Autodesk Inventor part; units mm, degrees
(part 2 of 2)
  arc A608 (10.5835, 25.1123) -> (10.4066, 24.8539) centre (14.8434, 22.0065) ccw
  arc A609 (10.8252, 25.4234) -> (10.5835, 25.1123) centre (15.7615, 21.3378) ccw
  arc A610 (11.147, 25.7878) -> (10.8252, 25.4234) centre (16.6706, 20.5861) ccw
  arc A611 (9.9958, 26.1618) -> (9.6113, 26.2702) centre (4.2393, 6.4866) ccw
  arc A612 (10.0419, 25.6779) -> (9.9958, 26.1618) centre (2.4697, 25.2002) ccw
  arc A613 (10.0547, 25.2841) -> (10.0419, 25.6779) centre (3.647, 25.2741) ccw
  arc A614 (10.4066, 24.8539) -> (10.0459, 24.9711) centre (4.2393, 6.4866) ccw
  arc A615 (10.0459, 24.9711) -> (10.0547, 25.2841) centre (4.7827, 25.2754) ccw
  arc A616 (9.1026, 25.5526) -> (8.9465, 25.2811) centre (13.5931, 22.7906) ccw
  arc A617 (9.3192, 25.8817) -> (9.1026, 25.5526) centre (14.5608, 22.1961) ccw
  arc A618 (9.6113, 26.2702) -> (9.3192, 25.8817) centre (15.526, 21.5179) ccw
  arc A619 (8.4344, 26.5528) -> (8.0426, 26.6307) centre (4.2393, 6.4866) ccw
  arc A620 (8.5183, 26.074) -> (8.4344, 26.5528) centre (1.0069, 25.0037) ccw
  arc A621 (8.5619, 25.6824) -> (8.5183, 26.074) centre (2.1747, 25.1697) ccw
  arc A622 (8.9465, 25.2811) -> (8.5777, 25.3697) centre (4.2393, 6.4866) ccw
  arc A623 (8.5777, 25.3697) -> (8.5619, 25.6824) centre (3.3069, 25.2601) ccw
  arc A624 (7.5917, 25.8754) -> (7.4574, 25.5925) centre (12.285, 23.4742) ccw
  arc A625 (7.7818, 26.2205) -> (7.5917, 25.8754) centre (13.2964, 22.9575) ccw
  arc A626 (8.0426, 26.6307) -> (7.7818, 26.2205) centre (14.3119, 22.3571) ccw
  arc A627 (6.8471, 26.8201) -> (6.4504, 26.867) centre (4.2393, 6.4866) ccw
  arc A628 (6.9683, 26.3493) -> (6.8471, 26.8201) centre (-0.436, 24.693) ccw
  arc A629 (7.0425, 25.9624) -> (6.9683, 26.3493) centre (0.7152, 24.9501) ccw
  arc A630 (7.4574, 25.5925) -> (7.0828, 25.6518) centre (4.2393, 6.4866) ccw
  arc A631 (7.0828, 25.6518) -> (7.0425, 25.9624) centre (1.8368, 25.1291) ccw
  arc A632 (6.0601, 26.0787) -> (5.9484, 25.7861) centre (10.9274, 24.0531) ccw
  arc A633 (6.2226, 26.4376) -> (6.0601, 26.0787) centre (11.9762, 23.6173) ccw
  arc A634 (6.4504, 26.867) -> (6.2226, 26.4376) centre (13.0356, 23.0985) ccw
  arc A635 (5.2437, 26.962) -> (4.8445, 26.9777) centre (4.2393, 6.4866) ccw
  arc A636 (5.4015, 26.5022) -> (5.2437, 26.962) centre (-1.85, 24.27) ccw
  arc A637 (5.5058, 26.1223) -> (5.4015, 26.5022) centre (-0.7225, 24.6167) ccw
  arc A638 (5.9484, 25.7861) -> (5.5703, 25.8158) centre (4.2393, 6.4866) ccw
  arc A639 (5.5703, 25.8158) -> (5.5058, 26.1223) centre (0.3816, 24.8831) ccw
  circle A640 centre (-6.2776, 14.9509) radius 1.5
  circle A641 centre (-6.2776, 14.9509) radius 3.5
  circle A642 centre (-4.225, -4.0303) radius 3.5
  circle A643 centre (-4.225, -4.0303) radius 1.5
  circle A644 centre (14.7563, -1.9776) radius 3.5
  circle A645 centre (14.7563, -1.9776) radius 1.5
  circle A646 centre (12.7036, 17.0036) radius 3.5
  circle A647 centre (12.7036, 17.0036) radius 1.5
  line L0 (-2.9801, 19.468) -> (-3.0512, 19.5957)
  circle A648 centre (4.2393, 6.4866) radius 5
  circle A649 centre (4.2393, 6.4866) radius 5.6
  circle A650 centre (4.2393, 6.4866) radius 18.25
  point P0 (0, 0)
  point P1 (4.2393, 28.9866)
  point P2 (2.474, 28.9173)
  point P3 (0.7195, 28.7096)
  point P4 (-1.0132, 28.3649)
  point P5 (-2.7136, 27.8854)
  point P6 (-4.3711, 27.2739)
  point P7 (-5.9755, 26.5343)
  point P8 (-7.5169, 25.671)
  point P9 (-8.9859, 24.6895)
  point P10 (-10.3733, 23.5958)
  point P11 (-11.6706, 22.3965)
  point P12 (-12.8698, 21.0992)
  point P13 (-13.9636, 19.7118)
  point P14 (-14.9451, 18.2428)
  point P15 (-15.8083, 16.7014)
  point P16 (-16.548, 15.097)
  point P17 (-17.1595, 13.4395)
  point P18 (-17.639, 11.7391)
  point P19 (-17.9837, 10.0064)
  point P20 (-18.1913, 8.252)
  point P21 (-18.2607, 6.4866)
  point P22 (-18.1913, 4.7213)
  point P23 (-17.9837, 2.9668)
  point P24 (-17.639, 1.2341)
  point P25 (-17.1595, -0.4663)
  point P26 (-16.548, -2.1238)
  point P27 (-15.8083, -3.7282)
  point P28 (-14.9451, -5.2696)
  point P29 (-13.9636, -6.7385)
  point P30 (-12.8698, -8.126)
  point P31 (-11.6706, -9.4233)
  point P32 (-10.3733, -10.6225)
  point P33 (-8.9859, -11.7163)
  point P34 (-7.5169, -12.6978)
  point P35 (-5.9755, -13.561)
  point P36 (-4.3711, -14.3007)
  point P37 (-2.7136, -14.9121)
  point P38 (-1.0132, -15.3917)
  point P39 (0.7195, -15.7364)
  point P40 (2.474, -15.944)
  point P41 (4.2393, -16.0134)
  point P42 (6.0046, -15.944)
  point P43 (7.7591, -15.7364)
  point P44 (9.4918, -15.3917)
  point P45 (11.1922, -14.9121)
  point P46 (12.8497, -14.3007)
  point P47 (14.4541, -13.561)
  point P48 (15.9955, -12.6978)
  point P49 (17.4645, -11.7163)
  point P50 (18.8519, -10.6225)
  point P51 (20.1492, -9.4233)
  point P52 (21.3484, -8.126)
  point P53 (22.4422, -6.7385)
  point P54 (23.4237, -5.2696)
  point P55 (24.287, -3.7282)
  point P56 (25.0266, -2.1238)
  point P57 (25.6381, -0.4663)
  point P58 (26.1176, 1.2341)
  point P59 (26.4623, 2.9668)
  point P60 (26.6699, 4.7213)
  point P61 (26.7393, 6.4866)
  point P62 (26.6699, 8.252)
  point P63 (26.4623, 10.0064)
  point P64 (26.1176, 11.7391)
  point P65 (25.6381, 13.4395)
  point P66 (25.0266, 15.097)
  point P67 (24.287, 16.7014)
  point P68 (23.4237, 18.2428)
  point P69 (22.4422, 19.7118)
  point P70 (21.3484, 21.0992)
  point P71 (20.1492, 22.3965)
  point P72 (18.8519, 23.5958)
  point P73 (17.4645, 24.6895)
  point P74 (15.9955, 25.671)
  point P75 (14.4541, 26.5343)
  point P76 (12.8497, 27.2739)
  point P77 (11.1922, 27.8854)
  point P78 (9.4918, 28.3649)
  point P79 (7.7591, 28.7096)
  point P80 (6.0046, 28.9173)
  point P81 (23.6134, 6.6762)
  point P82 (23.9112, 6.7638)
  point P83 (24.2822, 6.8975)
  point P84 (24.7304, 7.0918)
  point P85 (24.7147, 7.491)
  point P86 (24.2526, 7.6495)
  point P87 (23.8723, 7.7538)
  point P88 (23.5685, 7.8177)
  point P89 (23.5388, 8.1957)
  point P90 (23.8288, 8.3064)
  point P91 (24.1882, 8.4688)
  point P92 (24.6197, 8.6977)
  point P93 (24.5728, 9.0944)
  point P94 (24.0997, 9.2162)
  point P95 (23.7123, 9.2902)
  point P96 (23.4045, 9.3301)
  point P97 (23.3452, 9.7047)
  point P98 (23.6256, 9.8377)
  point P99 (23.9711, 10.0279)
  point P100 (24.3834, 10.2899)
  point P101 (24.3055, 10.6817)
  point P102 (23.8243, 10.766)
  point P103 (23.4323, 10.8094)
  point P104 (23.1223, 10.825)
  point P105 (23.0338, 11.1938)
  point P106 (23.3029, 11.3484)
  point P107 (23.6325, 11.5651)
  point P108 (24.0229, 11.8587)
  point P109 (23.9145, 12.2431)
  point P110 (23.4282, 12.2894)
  point P111 (23.034, 12.302)
  point P112 (22.7237, 12.2932)
  point P113 (22.6065, 12.6539)
  point P114 (22.8627, 12.8292)
  point P115 (23.1742, 13.071)
  point P116 (23.5404, 13.3943)
  point P117 (23.4022, 13.7691)
  point P118 (22.9138, 13.7771)
  point P119 (22.5198, 13.7587)
  point P120 (22.2112, 13.7256)
  point P121 (22.0661, 14.076)
  point P122 (22.3077, 14.2708)
  point P123 (22.5993, 14.5363)
  point P124 (22.939, 14.8874)
  point P125 (22.7717, 15.2501)
  point P126 (22.2842, 15.2198)
  point P127 (21.8929, 15.1705)
  point P128 (21.5878, 15.1133)
  point P129 (21.4156, 15.4512)
  point P130 (21.6413, 15.6644)
  point P131 (21.9111, 15.952)
  point P132 (22.2222, 16.3286)
  point P133 (22.027, 16.6771)
  point P134 (21.5434, 16.6086)
  point P135 (21.1571, 16.5288)
  point P136 (20.8575, 16.4479)
  point P137 (20.6593, 16.7712)
  point P138 (20.8675, 17.0015)
  point P139 (21.114, 17.3094)
  point P140 (21.3946, 17.7092)
  point P141 (21.1727, 18.0413)
  point P142 (20.6959, 17.9351)
  point P143 (20.3171, 17.8252)
  point P144 (20.0247, 17.721)
  point P145 (19.8018, 18.0278)
  point P146 (19.9913, 18.2737)
  point P147 (20.2128, 18.6)
  point P148 (20.4612, 19.0206)
  point P149 (20.2139, 19.3343)
  point P150 (19.7469, 19.191)
  point P151 (19.3779, 19.0517)
  point P152 (19.0946, 18.9249)
  point P153 (18.8483, 19.2133)
  point P154 (19.0179, 19.4732)
  point P155 (19.2132, 19.8159)
  point P156 (19.4278, 20.2547)
  point P157 (19.1566, 20.548)
  point P158 (18.7023, 20.3685)
  point P159 (18.3454, 20.2008)
  point P160 (18.0729, 20.0521)
  point P161 (17.8048, 20.3202)
  point P162 (17.9535, 20.5927)
  point P163 (18.1212, 20.9496)
  point P164 (18.3007, 21.4039)
  point P165 (18.0074, 21.6751)
  point P166 (17.5686, 21.4605)
  point P167 (17.2259, 21.2652)
  point P168 (16.966, 21.0956)
  point P169 (16.6776, 21.3419)
  point P170 (16.8044, 21.6252)
  point P171 (16.9436, 21.9942)
  point P172 (17.087, 22.4612)
  point P173 (16.7733, 22.7085)
  point P174 (16.3527, 22.4601)
  point P175 (16.0264, 22.2386)
  point P176 (15.7805, 22.0491)
  point P177 (15.4737, 22.272)
  point P178 (15.5779, 22.5644)
  point P179 (15.6878, 22.9432)
  point P180 (15.794, 23.42)
  point P181 (15.4619, 23.6419)
  point P182 (15.0621, 23.3613)
  point P183 (14.7541, 23.1148)
  point P184 (14.5239, 22.9067)
  point P185 (14.2006, 23.1048)
  point P186 (14.2815, 23.4045)
  point P187 (14.3613, 23.7907)
  point P188 (14.4298, 24.2743)
  point P189 (14.0813, 24.4695)
  point P190 (13.7047, 24.1584)
  point P191 (13.4171, 23.8886)
  point P192 (13.2039, 23.663)
  point P193 (12.866, 23.8351)
  point P194 (12.9232, 24.1402)
  point P195 (12.9724, 24.5315)
  point P196 (13.0028, 25.0191)
  point P197 (12.64, 25.1863)
  point P198 (12.289, 24.8466)
  point P199 (12.0235, 24.555)
  dimension "d2" = 360
  dimension "d10" = 3
  dimension "d11" = 7
  dimension "d14" = 360
  dimension "d30" = 10
  dimension "d31" = 0.6
  dimension "d42" = 36.5
  constraints: 1281 point on circle, 651 centre point, 8 coincident, 2 end point, 2656 other
  measures "d10" diameter of A640
  measures "d11" diameter of A641
  measures "d30" diameter of A648
  measures "d31" radial gap between concentric circles of A648 A649
  measures "d42" diameter of A650
extrude "押し出し1" add sketch "スケッチ1" along normal blind 3 contours A1 A2 A635 A636 A637 A639 A638 A632 A633 A634 A627 A628 A629 A631 A630 A624 A625 A626 A619 A620 A621 A623 A622 A616 A617 A618 A611 A612 A613 A615 A614 A608 A609 A610 A603 A604 A605 A607 A606 A600 A601 A602 A595 A596 A597 A599 A598 A592 A593 A594 A587 A588 A589 A591 A590 A584 A585 A586 A579 A580 A581 A583 A582 A576 A577 A578 A571 A572 A573 A575 A574 A568 A569 A570 A563 A564 A565 A567 A566 A560 A561 A562 A555 A556 A557 A559 A558 A552 A553 A554 A547 A548 A549 A551 A550 A544 A545 A546 A539 A540 A541 A543 A542 A536 A537 A538 A531 A532 A533 A535 A534 A528 A529 A530 A523 A524 A525 A527 A526 A520 A521 A522 A515 A516 A517 A519 A518 A512 A513 A514 A507 A508 A509 A511 A510 A504 A505 A506 A499 A500 A501 A503 A502 A496 A497 A498 A491 A492 A493 A495 A494 A488 A489 A490 A483 A484 A485 A487 A486 A480 A481 A482 A475 A476 A477 A479 A478 A472 A473 A474 A467 A468 A469 A471 A470 A464 A465 A466 A459 A460 A461 A463 A462 A456 A457 A458 A451 A452 A453 A455 A454 A448 A449 A450 A443 A444 A445 A447 A446 A440 A441 A442 A435 A436 A437 A439 A438 A432 A433 A434 A427 A428 A429 A431 A430 A424 A425 A426 A419 A420 A421 A423 A422 A416 A417 A418 A411 A412 A413 A415 A414 A408 A409 A410 A403 A404 A405 A407 A406 A400 A401 A402 A395 A396 A397 A399 A398 A392 A393 A394 A387 A388 A389 A391 A390 A384 A385 A386 A379 A380 A381 A383 A382 A376 A377 A378 A371 A372 A373 A375 A374 A368 A369 A370 A363 A364 A365 A367 A366 A360 A361 A362 A355 A356 A357 A359 A358 A352 A353 A354 A347 A348 A349 A351 A350 A344 A345 A346 A339 A340 A341 A343 A342 A336 A337 A338 A331 A332 A333 A335 A334 A328 A329 A330 A323 A324 A325 A327 A326 A320 A321 A322 A315 A316 A317 A319 A318 A312 A313 A314 A307 A308 A309 A311 A310 A304 A305 A306 A299 A300 A301 A303 A302 A296 A297 A298 A291 A292 A293 A295 A294 A288 A289 A290 A283 A284 A285 A287 A286 A280 A281 A282 A275 A276 A277 A279 A278 A272 A273 A274 A267 A268 A269 A271 A270 A264 A265 A266 A259 A260 A261 A263 A262 A256 A257 A258 A251 A252 A253 A255 A254 A248 A249 A250 A243 A244 A245 A247 A246 A240 A241 A242 A235 A236 A237 A239 A238 A232 A233 A234 A227 A228 A229 A231 A230 A224 A225 A226 A219 A220 A221 A223 A222 A216 A217 A218 A211 A212 A213 A215 A214 A208 A209 A210 A203 A204 A205 A207 A206 A200 A201 A202 A195 A196 A197 A199 A198 A192 A193 A194 A187 A188 A189 A191 A190 A184 A185 A186 A179 A180 A181 A183 A182 A176 A177 A178 A171 A172 A173 A175 A174 A168 A169 A170 A163 A164 A165 A167 A166 A160 A161 A162 A155 A156 A157 A159 A158 A152 A153 A154 A147 A148 A149 A151 A150 A144 A145 A146 A139 A140 A141 A143 A142 A136 A137 A138 A131 A132 A133 A135 A134 A128 A129 A130 A123 A124 A125 A127 A126 A120 A121 A122 A115 A116 A117 A119 A118 A112 A113 A114 A107 A108 A109 A111 A110 A104 A105 A106 A99 A100 A101 A103 A102 A96 A97 A98 A91 A92 A93 A95 A94 A88 A89 A90 A83 A84 A85 A87 A86 A80 A81 A82 A75 A76 A77 A79 A78 A72 A73 A74 A67 A68 A69 A71 A70 A64 A65 A66 A59 A60 A61 A63 A62 A56 A57 A58 A51 A52 A53 A55 A54 A48 A49 A50 A43 A44 A45 A47 A46 A40 A41 A42 A35 A36 A37 A39 A38 A32 A33 A34 A27 A28 A29 A31 A30 A24 A25 A26 A19 A20 A21 A23 A22 A16 A17 A18 A11 A12 A13 A15 A14 A8 A9 A10 A7 A5 A4 A3 A6 A0 | A641 | A642 | A644 | A646 | A649 | A650
extrude "押し出し7" cut sketch "スケッチ1" along normal blind 0.8 contours A641 | A642 | A644 | A646
extrude "押し出し8" cut sketch "スケッチ1" along normal blind 1.6 contours A649
